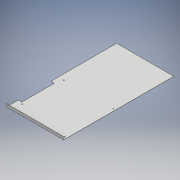
# Autodesk Inventor part: my trunk
Saved by Autodesk Inventor 2018 (Build 220112000, 112)
## iProperties
Created: 2018-06-19
Part Number: my trunk
Material: Generic
Document SubType Name: Sheet Metal
Designer: John Viljoen
Density: 1 g/cm^3
Sheet Metal Rule: Default_mm
Appearance: Default
Author: John Viljoen
Autodesk Inventor part; units mm, degrees
ref_plane "YZ Plane" through (0, 0, 0) normal (1, 0, 0) x (0, 1, 0)
ref_plane "XZ Plane" through (0, 0, 0) normal (0, 1, 0) x (-1, 0, 0)
ref_plane "XY Plane" through (0, 0, 0) normal (0, 0, 1) x (1, 0, 0)
sketch "Sketch1" plane through (0, 0, 0) normal (0, 0, 1) x (1, 0, 0)
  line L0 (0, 0) -> (181.174, 0)
  line L1 (181.174, 0) -> (181.174, 350.17)
  line L2 (181.174, 350.17) -> (0, 350.17)
  line L3 (0, 350.17) -> (0, 0)
  dimension "d0" = 181.174
  dimension "d1" = 350.17
  measures "d0" distance of L2.end L1.end
  measures "d1" distance of L1.end L0.end
extrude "Plate1" add sketch "Sketch1" along normal blind 0.5
sketch "Sketch3" plane through (181.174, 0.5, 0) normal (0, -1, 0) x (1, 0, 0)
  line L0 (-181.174, 0) -> (0, 0)
  line L1 (0, 0) -> (0, 10)
  line L2 (0, 10) -> (-181.174, 10)
  line L3 (-181.174, 10) -> (-181.174, 0)
  constraints: 6 end point, 1 horizontal, 1 perpendicular, 1 vertical
edge flange "Flange1" height 10 angle 90 thickness 0.5 bend radius 0.5 thickness toward (0, -1, 0) relief tear relief width 0.5 relief depth 0.25 edges at (90.587, 0, 0.5) wall of the first edge with corners at (0, 0.5, 0) (181.174, 0.5, 0) (181.174, 0.5, 10) (0, 0.5, 10)
bend "Bend1"
corner "Corner1"
sketch "Sketch4" plane through (0, 0, 0.5) normal (0, 0, 1) x (1, 0, 0)
  line L0 (181.174, 350.17) -> (181.174, 1) projected
  line L1 (10.4326, 171.5141) -> (10.4326, 6.5941)
  arc A0 (10.4326, 6.5941) -> (12.9726, 4.0541) centre (12.9726, 6.5941) ccw
  line L2 (177.8926, 4.0541) -> (12.9726, 4.0541)
  arc A1 (177.8926, 4.0541) -> (180.4326, 6.5941) centre (177.8926, 6.5941) ccw
  line L3 (180.4326, 171.5141) -> (180.4326, 6.5941)
  arc A2 (180.4326, 171.5141) -> (177.8926, 174.0541) centre (177.8926, 171.5141) ccw
  line L4 (177.8926, 174.0541) -> (12.9726, 174.0541)
  arc A3 (12.9726, 174.0541) -> (10.4326, 171.5141) centre (12.9726, 171.5141) ccw
  circle A4 centre (174.0826, 14.2141) radius 2.032
  circle A5 centre (174.0826, 169.1541) radius 2.032
  circle A6 centre (16.6026, 169.1541) radius 2.032
  circle A7 centre (16.6026, 37.0741) radius 2.032
  line L5 (181.174, 0) -> (181.174, 10.5)
  line L6 (181.174, 1) -> (181.174, 350.17) projected
  line L7 (181.174, 10.5) -> (174.824, 10.5) construction
  circle A8 centre (174.824, 10.5) radius 1.5
  line L8 (174.824, 10.5) -> (17.344, 10.5) construction
  line L9 (17.344, 10.5) -> (17.344, 33.36) construction
  circle A9 centre (17.344, 33.36) radius 1.5
  line L10 (17.344, 33.36) -> (17.344, 165.44) construction
  circle A10 centre (17.344, 165.0277) radius 1.5
  line L11 (174.824, 10.5) -> (174.824, 165.44) construction
  circle A11 centre (174.824, 165.44) radius 1.5
  point P0 (0, 0)
  point P1 (95.4326, 89.0541)
  dimension "d26" = 10.5
  dimension "d27" = 6.35
  dimension "d28" = 3
  dimension "d29" = 157.48
  dimension "d30" = 22.86
  dimension "d31" = 3
  dimension "d32" = 132.08
  dimension "d33" = 3
  dimension "d34" = 154.94
  dimension "d35" = 3
  constraints: 20 end point, 12 centre point, 8 point on circle, 3 coincident, 2 perpendicular, 2 point on line, 2 vertical, 1 horizontal
  measures "d26" distance of L5.start L5.end
  measures "d27" distance of L5.end L7.end
  measures "d28" diameter of A8
  measures "d29" distance of L8.start L8.end
  measures "d30" distance of L8.end L9.end
  measures "d31" diameter of A9
  measures "d32" distance of L10.start L10.end
  measures "d33" diameter of A10
  measures "d34" distance of L8.start L11.end
  measures "d35" diameter of A11
extrude "Extrusion2" cut sketch "Sketch4" against normal blind 10 contours A8 | A9 | A10 | A11
sketch "Sketch5" plane through (0, 0, 0.5) normal (0, 0, 1) x (1, 0, 0)
  circle A0 centre (17.344, 165.0277) radius 1.5 projected
  line L0 (0, 1) -> (0, 350.17) projected
  line L1 (17.344, 165.0277) -> (17.344, 131.5227) construction
  line L2 (17.344, 131.5227) -> (17.344, 43.5207) construction
  line L3 (17.344, 131.5227) -> (10.994, 131.5227) construction
  line L4 (10.994, 131.5227) -> (0, 131.5227)
  line L5 (0, 131.5227) -> (0, 43.5207)
  line L6 (0, 43.5207) -> (10.994, 43.5207)
  line L7 (10.994, 43.5207) -> (10.994, 131.5227)
  line L8 (10.994, 131.5227) -> (0, 131.5227)
  line L9 (0, 131.5227) -> (0, 141.5227)
  line L10 (0, 141.5227) -> (10.994, 141.5227)
  line L11 (10.994, 141.5227) -> (10.994, 131.5227)
  line L12 (0, 43.5207) -> (10.994, 43.5207)
  line L13 (10.994, 43.5207) -> (10.994, 38.5207)
  line L14 (10.994, 38.5207) -> (0, 38.5207)
  line L15 (0, 38.5207) -> (0, 43.5207)
  point P0 (0, 0)
  dimension "d38" = 33.505
  dimension "d39" = 88.002
  dimension "d40" = 6.35
  dimension "d43" = 10
  dimension "d44" = 5
  constraints: 30 end point, 6 parallel, 4 horizontal, 4 point on line, 3 perpendicular, 1 vertical
  measures "d38" distance of L1.start L1.end
  measures "d39" distance of L1.end L2.end
  measures "d40" distance of L1.end L3.end
  measures "d43" distance of L8.end L9.end
  measures "d44" distance of L12.end L13.end
extrude "Extrusion4" cut sketch "Sketch5" against normal blind 10 contours L0 L6 L13 L14 | L0 L4 L7 L6 | L0 L10 L11 L4
equation "\"d2\" = Thickness"
equation "\"d16\" = BendReliefWidth"
equation "\"d17\" = BendReliefDepth"
equation "\"d18\" = MinimumRemnant"
equation "\"d19\" = TransitionRadius"
equation "\"d22\" = BendRadius"
equation "\"d23\" = CornerReliefSize"
equation "\"d24\" = GapSize"
equation "\"d25\" = JacobiRadiusSize"
equation "\"BendRadius\" = Thickness"
equation "\"BendReliefWidth\" = Thickness"
equation "\"BendReliefDepth\" = 0.5 * Thickness"
equation "\"CornerReliefSize\" = 4 * Thickness"
equation "\"MinimumRemnant\" = 2 * Thickness"
equation "\"TransitionRadius\" = BendRadius"
equation "\"JacobiRadiusSize\" = BendRadius"
equation "\"GapSize\" = Thickness"
equation "\"Thickness\" = 0.5"
body "Solid1"
